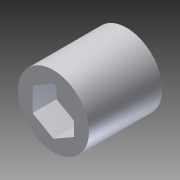
# Autodesk Inventor part: ServoToScrewKey
Saved by Autodesk Inventor 2012 (Build 160160000, 160)
## iProperties
Created: 2011-09-20
Part Number: ServoToScrewKey
Material: ABS Plastic
Document SubType Name: Modeling
Designer: KuttaA
Density: 1.06 g/cm^3
Mass: 4.22212 g
Surface Area: 27.1091 cm^2
Volume: 3.98313 cm^3
Author: KuttaA
Autodesk Inventor part; units mm, degrees
sketch "Sketch2" plane through (0, 0, 0) normal (0, 0, 1) x (1, 0, 0)
  circle A0 centre (0, 0) radius 10.3923
  line L0 (-4.0415, -7) -> (4.0415, -7) projected
  line L1 (4.0415, -7) -> (8.0829, 0) projected
  line L2 (8.0829, 0) -> (4.0415, 7) projected
  line L3 (4.0415, 7) -> (-4.0415, 7) projected
  line L4 (-4.0415, 7) -> (-8.0829, 0) projected
  line L5 (-8.0829, 0) -> (-4.0415, -7) projected
  line L6 (4.0415, 7) -> (5.1962, 9) construction
  line L7 (-8.3716, 0) -> (-4.1858, -7.25)
  line L8 (-4.1858, -7.25) -> (4.1858, -7.25)
  line L9 (4.1858, -7.25) -> (8.3716, 0)
  line L10 (8.3716, 0) -> (4.1858, 7.25)
  line L11 (4.1858, 7.25) -> (-4.1858, 7.25)
  line L12 (-4.1858, 7.25) -> (-8.3716, 0)
  dimension "d9" = 2
  dimension "d10" = 0.25
  dimension "d11" = 0.25
  dimension "d12" = 0.25
  dimension "d13" = 0.25
  dimension "d14" = 0.25
  dimension "d15" = 0.25
  constraints: 14 end point, 7 parallel, 1 coincident, 3 other
  measures "d9" vertical distance of L2.end L6.end
  measures "d10" distance between parallel lines of L4 L12
  measures "d11" distance between parallel lines of L11 L3
  measures "d12" distance between parallel lines of L10 L2
  measures "d13" distance between parallel lines of L9 L1
  measures "d14" distance between parallel lines of L8 L0
  measures "d15" distance between parallel lines of L7 L5
ref_plane "Work Plane1" through (-12.7, 0, -12.7) normal (0, 0, 1) x (1, 0, 0)
ref_plane "Work Plane2" through (-11.7, 1, -12.7) normal (0, 0, 1) x (1, 0, 0)
ref_plane "Work Plane3" through (-8.125, -8.125, -9.7) normal (0, 0, 1) x (1, 0, 0)
extrude "Extrusion3" add sketch "Sketch2" against normal up to surface (9.7 mm away) contours A0
sketch "Sketch4" plane through (0, 0, 0) normal (0, 0, 1) x (1, 0, 0)
  circle A0 centre (0, 0) radius 10.3923 projected
extrude "Extrusion4" add sketch "Sketch4" along normal blind 12
sketch "Sketch5" plane through (0, 0, -9.7) normal (0, 0, -1) x (-1, 0, 0)
  circle A0 centre (0, 0) radius 10.3923 projected
  point P0 (0, 0)
extrude "Extrusion5" cut sketch "Sketch5" against normal blind 0.3
sketch "Sketch6" plane through (0, 0, 12) normal (0, 0, 1) x (1, 0, 0)
  line L0 (-6.05, 3.493) -> (0, 6.9859)
  line L1 (0, 6.9859) -> (6.05, 3.493)
  line L2 (6.05, 3.493) -> (6.05, -3.493)
  line L3 (6.05, -3.493) -> (0, -6.9859)
  line L4 (0, -6.9859) -> (-6.05, -3.493)
  line L5 (-6.05, -3.493) -> (-6.05, 3.493)
  line L6 (-14.5492, 0) -> (14.5492, 0) projected
  line L7 (0, -6.9859) -> (0, 6.9859) construction
  line L8 (6.05, -3.493) -> (-6.05, 3.493) construction
  line L9 (0, -14.5492) -> (0, 14.5492) projected
  point P0 (0, 0)
  point P1 (14.5492, 0)
  point P2 (0, 0)
  dimension "d32" = 0
  dimension "d35" = 12.1
  constraints: 16 end point, 4 equal length, 4 parallel, 1 coincident, 1 midpoint, 1 other
  measures "d32" distance between parallel lines of L9 L7
  measures "d35" distance between parallel lines of L2 L5
extrude "Extrusion6" cut sketch "Sketch6" against normal blind 7
sketch "Sketch7" plane through (0, 0, 5) normal (0, 0, 1) x (1, 0, 0)
  circle A0 centre (0, 0) radius 2.15
  point P0 (0, 0)
  dimension "d21" = 4.3
  constraints: 1 centre point, 1 coincident
  measures "d21" diameter of A0
extrude "Extrusion7" cut sketch "Sketch7" against normal through all
sketch "Sketch10" plane through (0, 0, 0) normal (0, 0, -1) x (-1, 0, 0)
  circle A0 centre (0, 0) radius 10.3923 projected
  circle A1 centre (0, 0) radius 4.5
  dimension "d25" = 9
  constraints: 1 centre point, 1 coincident
  measures "d25" diameter of A1
extrude "Extrusion8" cut sketch "Sketch10" against normal blind 1 contours A1
equation "\"d11\" = d10"
equation "\"d12\" = d11"
equation "\"d13\" = d12"
equation "\"d14\" = d13"
equation "\"d15\" = d14"
body "Solid2"
